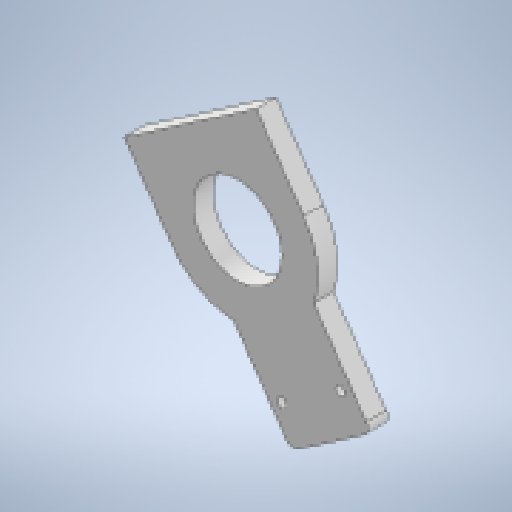
# Autodesk Inventor part: sukima
Saved by Autodesk Inventor 2024 (Build 280153000, 153)
## iProperties
Created: 2024-06-05
Part Number: sukima
Material: 一般
Document SubType Name: Modeling
Designer: right
Density: 1 g/cm^3
Appearance: 既定
Author: right
Autodesk Inventor part; units mm, degrees
ref_plane "YZ Plane" through (0, 0, 0) normal (1, 0, 0) x (0, 1, 0)
ref_plane "XZ Plane" through (0, 0, 0) normal (0, 1, 0) x (-1, 0, 0)
ref_plane "XY Plane" through (0, 0, 0) normal (0, 0, 1) x (1, 0, 0)
sketch "スケッチ1" plane through (0, 0, 0) normal (0, 0, 1) x (1, 0, 0)
  circle A0 centre (-0.5053, 0.7372) radius 6.2325 projected
  circle A1 centre (-0.5053, 0.7372) radius 10 projected
  circle A2 centre (-0.5053, 0.7372) radius 18.1063
  arc A3 (-9.248, 16.5929) -> (-9.2505, 16.5915) centre (-0.5053, 0.7372) ccw projected
  point P0 (0, 0)
  constraints: 1 coincident, 3 other
ref_plane "作業平面1" through (-13.4276, -31.9146, 4.5) normal (0, 0, -1) x (-0.5653297, 0.824865, 0)
extrude "押し出し1" add sketch "スケッチ1" along normal up to surface (4.5 mm away) contours A2
sketch "スケッチ2" plane through (-0.5053, 0.7372, 4.5) normal (0, 0, 1) x (1, 0, 0)
  line L0 (-41.2386, -0.38) -> (-20.4108, 13.8946) projected
  circle A0 centre (0, 0) radius 18.1063 projected
  line L1 (-25.6765, 5.4364) -> (4.1939, 25.9084)
  line L2 (-25.6765, 5.4364) -> (-13.3884, -12.4929)
  line L3 (4.1939, 25.9084) -> (14.9352, 10.236)
  circle A1 centre (0, 0) radius 10 projected
  point P0 (0.5053, -0.7372)
  point P1 (-10.236, 14.9352)
  point P2 (-14.9352, -10.236)
  dimension "d9" = 19
  constraints: 6 end point, 2 perpendicular, 1 parallel, 4 other
  measures "d9" distance from line of A1.centre L1
extrude "押し出し2" add sketch "スケッチ2" against normal up to surface (4.5 mm away) contours A0 L2 L1 L3
sketch "スケッチ3" plane through (-26.1817, 6.1737, 4.5) normal (0, 0, 1) x (0.824865, 0.5653297, 0)
  circle A0 centre (26.1063, -48.5) radius 1
  circle A1 centre (10.1063, -48.5) radius 1.05 construction
  circle A2 centre (26.1063, -48.5) radius 1.1
  circle A3 centre (10.1063, -48.5) radius 1.1
  line L0 (29.1063, -33.3818) -> (29.1063, -51.5)
  line L1 (29.1063, -51.5) -> (7.1063, -51.5)
  line L2 (7.1063, -51.5) -> (7.1063, -33.3818)
  circle A4 centre (26.1063, -48.5) radius 3
  arc A5 (0, -19) -> (36.2125, -19) centre (18.1063, -19) ccw projected
  circle A6 centre (10.1063, -48.5) radius 3
  circle A7 centre (26.1063, -48.5) radius 1.8 projected
  point P0 (18.1063, -19.8937)
  point P1 (10.1063, -51.5)
  point P2 (26.1063, -51.5)
  point P3 (29.1063, -48.5)
  point P4 (7.1063, -48.5)
  dimension "d4" = 2.2
  dimension "d5" = 2.2
  dimension "d6" = 6
  constraints: 6 centre point, 6 end point, 5 coincident, 4 tangent, 2 point on circle, 1 parallel, 1 perpendicular, 1 vertical
  measures "d4" diameter of A2
  measures "d5" diameter of A3
  measures "d6" diameter of A4
extrude "押し出し3" add sketch "スケッチ3" against normal up to surface (4.5 mm away) contours L0 A4 L1 A6 L2 A5 | A4 | A6 | A7
sketch "スケッチ4" plane through (0, 0, 0) normal (0, 0, -1) x (-1, 0, 0)
  line L0 (-25.2455, -17.3777) -> (-16.6987, -4.9072) projected
  line L1 (-25.2455, -17.3777) -> (-29.7681, -23.9766)
  line L2 (-29.7681, -23.9766) -> (-11.6211, -36.4138)
  line L3 (-11.6211, -36.4138) -> (-7.0984, -29.8149)
  line L4 (-24.4669, -21.5483) -> (-11.269, -30.5935) projected
  arc A0 (-25.2455, -17.3777) -> (-24.4669, -21.5483) centre (-22.7709, -19.0737) ccw projected
  arc A1 (-11.3877, -26.8752) -> (-7.4259, -27.6394) centre (-9.573, -28.1189) ccw projected
  arc A2 (-11.269, -30.5935) -> (-7.0984, -29.8149) centre (-9.573, -28.1189) ccw projected
  point P0 (0, 0)
  dimension "d10" = 5
  constraints: 6 end point, 1 coincident, 1 collinear, 1 parallel, 1 perpendicular
  measures "d10" distance between parallel lines of L4 L2
extrude "押し出し4" add sketch "スケッチ4" against normal up to surface (4.5 mm away)
fillet "フィレット1" radius 2 2 edges at (29.7681, -23.9766, 2.25) (11.6211, -36.4138, 2.25)
sketch "スケッチ5" plane through (0, 0, 0) normal (0, 0, -1) x (-1, 0, 0)
  circle A0 centre (-9.573, -28.1189) radius 1.1 projected
  circle A1 centre (-9.573, -28.1189) radius 2
  circle A2 centre (-22.7709, -19.0737) radius 1.1 projected
  circle A3 centre (-22.7709, -19.0737) radius 2
  point P0 (0, 0)
  dimension "d14" = 4
  dimension "d15" = 4
  constraints: 2 centre point, 2 coincident
  measures "d14" diameter of A1
  measures "d15" diameter of A3
extrude "押し出し5" cut sketch "スケッチ5" against normal blind 2 contours A0 | A1 | A2 | A3
sketch "スケッチ6" plane through (0, 0, 0) normal (0, 0, -1) x (-1, 0, 0)
  line L0 (-10.4904, -34.7641) -> (1.4483, -17.3445) projected
  line L1 (-8.7944, -32.2895) -> (-26.9415, -19.8523)
  line L2 (-16.6987, -4.9072) -> (-28.6375, -22.3269) projected
  line L3 (-28.1184, -25.1072) -> (-13.2708, -35.2832) projected
  arc A0 (-13.2708, -35.2832) -> (-10.4904, -34.7641) centre (-12.1402, -33.6335) ccw projected
  arc A1 (-28.6375, -22.3269) -> (-28.1184, -25.1072) centre (-26.9877, -23.4575) ccw projected
  point P0 (0, 0)
  dimension "d18" = 5
  constraints: 2 end point, 2 point on line
  measures "d18" distance between parallel lines of L3 L1
ref_plane "作業平面2" through (26.7732, -7.348, -3) normal (0, 0, -1) x (-0.5653297, 0.824865, 0)
extrude "押し出し6" add sketch "スケッチ6" along normal up to surface (3 mm away)
